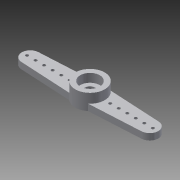
# Autodesk Inventor part: ServoBlade
Saved by Autodesk Inventor 2014 SP1 (Build 180222100, 222)
## iProperties
Created: 2017-01-16
Part Number: ServoBlade
Material: Generic
Document SubType Name: Modeling
Designer: danielsikar
Density: 1 g/cm^3
Appearance: Smooth - White
Author: danielsikar
Autodesk Inventor part; units mm, degrees
ref_plane "YZ Plane" through (0, 0, 0) normal (1, 0, 0) x (0, 1, 0)
ref_plane "XZ Plane" through (0, 0, 0) normal (0, 1, 0) x (-1, 0, 0)
ref_plane "XY Plane" through (0, 0, 0) normal (0, 0, 1) x (1, 0, 0)
sketch "Sketch1" plane through (0, 0, 0) normal (0, 0, 1) x (1, 0, 0)
  circle A0 centre (0, 0) radius 15.9 construction
  line L0 (-15.9, 2.9943) -> (-15.9, -4.6321) construction
  line L1 (15.9, 4.7345) -> (15.9, -4.6321) construction
  circle A1 centre (0, 0) radius 3.45 construction
  arc A2 (-14.1096, 1.997) -> (-14.1096, -1.997) centre (-14, 0) ccw
  arc A3 (14.1096, -1.997) -> (14.1096, 1.997) centre (14, 0) ccw
  line L2 (4.9743, 2.65) -> (-6.1832, 2.65) construction
  line L3 (-6.1832, 2.65) -> (-6.1832, -2.65) construction
  line L4 (-6.1832, -2.65) -> (4.9743, -2.65) construction
  line L5 (4.9743, -2.65) -> (4.9743, 2.65) construction
  line L6 (-2.2091, 2.65) -> (-14.1096, 1.997)
  line L7 (-2.2091, -2.65) -> (-14.1096, -1.997)
  line L8 (2.2091, 2.65) -> (14.1096, 1.997)
  line L9 (2.2091, -2.65) -> (14.1096, -1.997)
  line L10 (-18.8016, 0) -> (-15.9, 0) construction
  line L11 (-12, 0) -> (22.4015, 0) construction
  arc A4 (-2.2091, -2.65) -> (2.2091, -2.65) centre (0, 0) ccw
  arc A5 (2.2091, 2.65) -> (-2.2091, 2.65) centre (0, 0) ccw
  dimension "d0" = 31.8
  dimension "d1" = 6.9
  dimension "d4" = 4
  dimension "d5" = 4
  dimension "d6" = 14
  dimension "d7" = 14
  dimension "d8" = 5.3
  constraints: 24 end point, 8 point on circle, 6 centre point, 6 point on line, 4 tangent, 3 coincident, 3 horizontal, 3 parallel, 3 perpendicular
  measures "d0" diameter of A0
  measures "d1" diameter of A1
  measures "d4" diameter of A2
  measures "d5" diameter of A3
  measures "d6" distance of point (0, 0) A2.centre
  measures "d7" distance of A3.centre point (0, 0)
  measures "d8" distance of L3.end L2.end
extrude "Extrusion1" add sketch "Sketch1" along normal blind 1.5
sketch "Sketch2" plane through (0, 0, 1.5) normal (0, 0, 1) x (1, 0, 0)
  arc A0 (2.2091, 2.65) -> (-2.2091, 2.65) centre (0, 0) ccw projected
  circle A1 centre (0, 0) radius 3.45
  constraints: 1 centre point, 1 coincident
extrude "Extrusion2" add sketch "Sketch2" along normal blind 2.2
sketch "Sketch3" plane through (0, 0, 3.7) normal (0, 0, 1) x (1, 0, 0)
  circle A0 centre (0, 0) radius 3.45 projected
  circle A1 centre (0, 0) radius 2.3
  dimension "d12" = 4.6
  constraints: 1 centre point, 1 coincident
  measures "d12" diameter of A1
extrude "Extrusion3" cut sketch "Sketch3" against normal blind 2 contours A1
sketch "Sketch4" plane through (0, 0, 0) normal (0, 0, -1) x (-1, 0, 0)
  arc A0 (-2.2091, -2.65) -> (2.2091, -2.65) centre (0, 0) ccw projected
  circle A1 centre (0, 0) radius 2.3
  dimension "d15" = 4.6
  constraints: 1 centre point, 1 coincident
  measures "d15" diameter of A1
extrude "Extrusion4" cut sketch "Sketch4" against normal blind 1
sketch "Sketch5" plane through (0, 0, 1) normal (0, 0, -1) x (-1, 0, 0)
  circle A0 centre (0, 0) radius 2.3 projected
  circle A1 centre (0, 0) radius 1.25
  dimension "d18" = 2.5
  constraints: 1 centre point, 1 coincident
  measures "d18" diameter of A1
extrude "Extrusion5" cut sketch "Sketch5" against normal blind 1 contours A1
sketch "Sketch6" plane through (0, 0, 1.5) normal (0, 0, 1) x (1, 0, 0)
  circle A0 centre (14.7413, 0) radius 0.35
  dimension "d21" = 0.7
  constraints: 1 centre point
  measures "d21" diameter of A0
extrude "Extrusion6" cut sketch "Sketch6" against normal through all
pattern_linear "Rectangular Pattern1" count 6 spacing 2 along (-1, 0, 0) of "Extrusion6"
mirror "Mirror1" about plane through (0, 0, 0) normal (1, 0, 0) of "Extrusion6", "Rectangular Pattern1"
body "Solid1"
